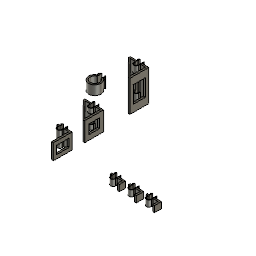
EinklickbareHalterungen (Autodesk Fusion 360 design; units mm, degrees)
part number: 2025-11-29-23-14-23-792
Autodesk Fusion 360 part; units mm, degrees
note: some values were not read from the file. Chosen so that the rebuilt part matches the saved one: which bodies a step acts on; which face or edge a step refers to. Set by a fixed rule: which sketch regions a step uses.
sketch "Skizze1" plane through (0, 0, 0) normal (0, 0, 1) x (1, 0, 0)
  line L0 (0, 0) -> (50, 0)
  line L1 (50, 0) -> (50, 25)
  line L2 (50, 25) -> (0, 25)
  line L3 (0, 25) -> (0, 0)
  line L4 (38.3, 22) -> (11.7, 22)
  line L5 (11.7, 22) -> (11.7, 3)
  line L6 (11.7, 3) -> (38.3, 3)
  line L7 (38.3, 3) -> (38.3, 22)
  line L8 (38.3, 22) -> (11.7, 3) construction
  line L9 (11.7, 22) -> (38.3, 3) construction
  point P0 (25, 12.5)
  dimension "d1" = 50
  dimension "d2" = 25
  dimension "d3" = 26.6
  dimension "d4" = 19
  constraint horizontal L0
  constraint vertical L1
  constraint horizontal L2
  constraint vertical L3
  constraint coincident L0.start L3.end
  constraint horizontal L4
  constraint perpendicular L4 L5
  constraint parallel L4 L6
  constraint parallel L5 L7
  constraint coincident L8 P0
  constraint coincident L9 P0
  measures "d1" distance of L0.start L0.end
  measures "d2" distance of L0.start L2.end
  measures "d3" distance of L5.end L6.end
  measures "d4" distance of L4.end L5.end
extrude "Extrusion1" add sketch "Skizze1" along normal blind 2 makes body 1
sketch "Skizze2" plane through (0, 0, 2) normal (0, 0, 1) x (-1, 0, 0)
  line L0 (-38.3, -22) -> (-38.3, -3)
  line L1 (-38.3, -3) -> (-11.7, -3)
  line L2 (-11.7, -3) -> (-11.7, -22)
  line L3 (-11.7, -22) -> (-38.3, -22)
  line L4 (0, -25) -> (0, 0)
  line L5 (0, 0) -> (-50, 0)
  line L6 (-50, 0) -> (-50, -25)
  line L7 (-50, -25) -> (0, -25)
  line L8 (-11.7, -12.5) -> (-5, -12.5)
  line L9 (-38.3, -12.5) -> (-45, -12.5)
  circle A0 centre (-5, -12.5) radius 1.35
  circle A1 centre (-45, -12.5) radius 1.35
  dimension "d7" = 6.7
  dimension "d8" = 6.7
  dimension "d9" = 2.7
  dimension "d10" = 2.7
  constraint midpoint L2 L8.start
  constraint perpendicular L0 L8
  constraint midpoint L0 L9.start
  constraint perpendicular L0 L9
  constraint coincident L8.end A0.centre
  constraint coincident L9.end A1.centre
  measures "d7" distance of L8.start L8.end
  measures "d8" distance of L9.start L9.end
  measures "d9" diameter of A0
  measures "d10" diameter of A1
sketch "Skizze3" plane through (0, 0, 0) normal (0, 1, 0) x (1, 0, 0)
sketch "Skizze4" plane through (0, 0, 2) normal (0, 0, 1) x (-1, 0, 0)
  line L0 (-38.3, -22) -> (-38.3, -3)
  line L1 (-38.3, -3) -> (-11.7, -3)
  line L2 (-11.7, -3) -> (-11.7, -22)
  line L3 (-11.7, -22) -> (-38.3, -22)
  line L4 (0, -25) -> (0, 0)
  line L5 (0, 0) -> (-50, 0)
  line L6 (-50, 0) -> (-50, -25)
  line L7 (-50, -25) -> (0, -25)
  line L8 (-110, 0) -> (-80, 0)
  line L9 (-80, 0) -> (-80, -25)
  line L10 (-80, -25) -> (-110, -25)
  line L11 (-110, -25) -> (-110, 0)
  dimension "d13" = 30
  dimension "d14" = 25
  constraint horizontal L8
  constraint vertical L9
  constraint horizontal L10
  constraint vertical L11
  measures "d13" distance of L8.start L8.end
  measures "d14" distance of L8.start L10.end
sketch "Skizze5" plane through (0, 0, 1) normal (0, 0, 1) x (-1, 0, 0)
  line L0 (-110, -25) -> (-80, -25)
  line L1 (-80, -25) -> (-80, 0)
  line L2 (-80, 0) -> (-110, 0)
  line L3 (-110, 0) -> (-110, -25)
  line L4 (-80, 0) -> (-110, -25) construction
  line L5 (-110, 0) -> (-80, -25) construction
  line L6 (-102.25, -20.5) -> (-87.75, -20.5)
  line L7 (-87.75, -20.5) -> (-87.75, -4.5)
  line L8 (-87.75, -4.5) -> (-102.25, -4.5)
  line L9 (-102.25, -4.5) -> (-102.25, -20.5)
  line L10 (-102.25, -20.5) -> (-87.75, -4.5) construction
  line L11 (-87.75, -20.5) -> (-102.25, -4.5) construction
  point P0 (-95, -12.5)
  dimension "d17" = 14.5
  dimension "d18" = 16
  constraint coincident L1.end L2.start
  constraint coincident L0.start L3.end
  constraint coincident L2.end L3.start
  constraint coincident L0.end L1.start
  constraint horizontal L6
  constraint perpendicular L6 L7
  constraint parallel L6 L8
  constraint parallel L7 L9
  constraint coincident L10 P0
  constraint coincident L11 P0
  constraint midpoint L4 P0
  measures "d17" distance of L7.end L8.end
  measures "d18" distance of L6.end L7.end
move_body "Verschieben2" [no effect]
sketch "Skizze6" plane through (0, 0, 0) normal (-1, 0, 0) x (0, -1, 0)
  line L0 (-25, 0) -> (0, 0)
  line L1 (0, 0) -> (0, 2)
  line L2 (0, 2) -> (-25, 2)
  line L3 (-25, 2) -> (-25, 0)
  line L4 (-25, 0) -> (-25, 10.9)
  line L5 (-25, 0) -> (-23.5, 0)
  line L6 (-23.5, 0) -> (-23.5, 30)
  line L7 (-23.5, 30) -> (-25, 30)
  line L8 (-25, 30) -> (-25, 0)
  line L9 (-25, 30) -> (-25, 19.1)
  line L10 (-25, 10.9) -> (-25, 11.9)
  line L11 (-25, 19.1) -> (-25, 18.1)
  line L12 (-25, 11.9) -> (-25, 18.1)
  line L13 (-25, 0) -> (-25, 11)
  line L14 (-25, 30) -> (-25, 19)
  line L15 (-25, 19) -> (-27.3, 19)
  line L16 (-27.3, 19) -> (-27.3, 20.5)
  line L17 (-25, 10.9) -> (-25, 11.65)
  line L18 (-27.3, 9.4) -> (-24.118, 9.4) construction
  line L19 (-25, 19) -> (-25, 18.25)
  line L20 (-27.3, 20.5) -> (-29.55, 18.25)
  line L21 (-27.3, 20.5) -> (-24.118, 20.5) construction
  line L22 (-29.55, 18.25) -> (-25, 18.25)
  line L23 (-25, 30) -> (-25, 22)
  line L24 (-25, 22) -> (-23.5, 22)
  line L25 (-25, 15) -> (-20, 15) construction
  line L26 (-25, 18.25) -> (-20, 18.25)
  line L27 (-25, 19) -> (-20, 19)
  line L28 (-25, 0) -> (-25, 11)
  line L29 (-25, 11) -> (-27.3, 11)
  line L30 (-27.3, 11) -> (-27.3, 9.5)
  line L31 (-25, 11) -> (-25, 11.75)
  line L32 (-27.3, 9.5) -> (-29.5511, 11.75)
  line L33 (-29.5511, 11.75) -> (-25, 11.75)
  circle A0 centre (-20, 15) radius 3.25
  line L34 (-25, 11) -> (-20, 11)
  line L35 (-25, 11.75) -> (-20, 11.75)
  circle A1 centre (-20, 15) radius 4
  dimension "d29" = 10.9
  dimension "d30" = 1.5
  dimension "d31" = 30
  dimension "d32" = 10.9
  dimension "d42" = 1
  dimension "d43" = 1
  dimension "d52" = 11
  dimension "d53" = 2.3
  dimension "d54" = 1.5
  dimension "d56" = 0.75
  dimension "d58" = 0.75
  dimension "d59" = 135
  dimension "d61" = 1.5
  dimension "d62" = 0.75
  constraint coincident L0.start L3.end
  constraint perpendicular L2 L4
  constraint horizontal L5
  constraint vertical L6
  constraint horizontal L7
  constraint vertical L8
  constraint perpendicular L7 L9
  constraint coincident L10 L13.end
  constraint parallel L10 L13
  constraint perpendicular L7 L14
  constraint perpendicular L14 L15
  constraint perpendicular L15 L16
  constraint horizontal L18
  constraint perpendicular L15 L19
  constraint horizontal L21
  constraint perpendicular L8 L22
  constraint coincident L14 L23.end
  constraint coincident L6 L24.end
  constraint perpendicular L6 L24
  constraint midpoint L12 L25.start
  constraint perpendicular L12 L25
  constraint perpendicular L11 L26
  constraint perpendicular L8 L27
  constraint perpendicular L16 L29
  constraint perpendicular L18 L30
  constraint perpendicular L29 L31
  constraint perpendicular L8 L33
  constraint coincident L25.end A0.centre
  constraint coincident L26.end A0
  constraint tangent L26 A0
  constraint perpendicular L17 L34
  constraint coincident A0 L35.end
  constraint tangent A0 L35
  constraint coincident L27.end A1
  constraint tangent L27 A1
  measures "d29" distance of L0.start L4.end
  measures "d30" distance of L0.start L5.end
  measures "d31" distance of L0.start L7.end
  measures "d32" distance of L7.end L9.end
  measures "d42" distance of L4.end L10.end
  measures "d43" distance of L9.end L11.end
  measures "d52" distance of L7.end L14.end
  measures "d53" distance of L14.end L15.end
  measures "d54" distance of L15.end L16.end
  measures "d56" distance of L4.end L17.end
  measures "d58" distance of L14.end L19.end
  measures "d59" angle of L20 L21
  measures "d61" distance of L29.end L30.end
  measures "d62" distance of L13.end L31.end
extrude "Extrusion12" add sketch "Skizze6" against normal blind 50 contours L2 L4 L6 L8 L10 L13 L17 L28 L34 | L6 L8 L10 L17 L31 L34 L35 | L6 L34 L35 A1 | L8 L10 L17 L29 L30 L31 L32 L33 | L26 A0 L35 A1 | L6 L26 L27 A1 | L6 L8 L11 L19 L26 L27 | L6 L8 L9 L11 L14 L24 L27 | L8 L11 L15 L16 L19 L20 L22 bodies 1
move_body "Verschieben5" bodies 1 to x (0, 0, 1) y (0, 1, 0) z (-1, 0, 0) at (0, 0, 0)
sketch "Skizze7" plane through (0, 0, 0) normal (0, 0, 1) x (1, 0, 0)
  circle A0 centre (55, 0) radius 7.5
  circle A1 centre (55, 0) radius 10
  line L0 (55, 0) -> (58, 0)
  line L1 (58, 0) -> (52, 0)
  line L2 (52, 0) -> (52, 20)
  line L3 (52, 20) -> (58, 20)
  line L4 (58, 20) -> (58, 0)
  line L5 (55, 0) -> (59.7, 0)
  line L6 (59.7, 0) -> (50.3, 0)
  line L7 (50.3, 0) -> (50.3, 20)
  line L8 (50.3, 20) -> (59.7, 20)
  line L9 (59.7, 20) -> (59.7, 0)
  line L10 (50.3, 8.8267) -> (50.3, 11.0767)
  line L11 (59.7, 8.8267) -> (59.7, 11.0767)
  line L12 (59.7, 11.0767) -> (61.38, 11.0767)
  line L13 (50.3, 11.0767) -> (48.62, 11.0767)
  line L14 (48.62, 11.0767) -> (52, 14.4567)
  line L15 (48.62, 11.0767) -> (53.4, 11.0767) construction
  line L16 (61.38, 11.0767) -> (58, 14.4567)
  dimension "d66" = 15
  dimension "d67" = 20
  dimension "d68" = 6
  dimension "d69" = 20
  dimension "d71" = 9.4
  dimension "d72" = 20
  dimension "d73" = 2.25
  dimension "d74" = 2.25
  dimension "d75" = 1.68
  dimension "d76" = 1.68
  dimension "d77" = 45
  constraint concentric A0 A1
  constraint coincident A0.centre A1.centre
  constraint horizontal L0
  constraint horizontal L1
  constraint vertical L2
  constraint horizontal L3
  constraint vertical L4
  constraint perpendicular L4 L5
  constraint horizontal L6
  constraint vertical L7
  constraint horizontal L8
  constraint vertical L9
  constraint coincident A1 L10.start
  constraint coincident L7 L10.start
  constraint parallel L7 L10
  constraint coincident A1 L11.start
  constraint coincident L9 L11.start
  constraint parallel L9 L11
  constraint perpendicular L11 L12
  constraint perpendicular L7 L13
  constraint horizontal L15
  constraint coincident L2 L14.end
  constraint coincident L4 L16.end
  constraint perpendicular L14 L16
  measures "d66" diameter of A0
  measures "d67" diameter of A1
  measures "d68" distance of L0.end L1.end
  measures "d69" distance of L1 L3
  measures "d71" distance of L5.end L6.end
  measures "d72" distance of L5.end L8.end
  measures "d73" distance of L10.start L10.end
  measures "d74" distance of L11.start L11.end
  measures "d75" distance of L11.end L12.end
  measures "d76" distance of L10.end L13.end
  measures "d77" angle of L14 L15
extrude "Extrusion13" add sketch "Skizze7" along normal blind 2 separate body contours A0 A1 L7 L9 | A0 A1 L4 L9 | A0 A1 L2 L7 | A1 L4 L9 L11 L16 | A1 L2 L7 L10 L14 | L9 L12 L16 | L7 L13 L14 makes body 2
extrude "Extrusion14" add 1 faces at (51.4333, 12.2509, 2) along direction (0, 0, 1) blind 3 on bodies 2 bodies 2
sketch "Skizze8" plane through (0, 0, 0) normal (0, 0, 1) x (1, 0, 0)
  line L0 (55, 0) -> (70, 0)
  line L1 (59.7, 8.8267) -> (59.7, 11.0767)
  arc A0 (50.3, 8.8267) -> (59.7, 8.8267) centre (55, 0) ccw
  line L2 (59.7, 8.8267) -> (70, 8.8267)
  line L3 (70, 8.8267) -> (70, -16.1733)
  line L4 (70, 8.8267) -> (68, 8.8267)
  line L5 (68, 8.8267) -> (68, -16.1733)
  line L6 (68, -16.1733) -> (70, -16.1733)
  line L7 (70, -16.1733) -> (70, 8.8267)
  line L8 (68, 0) -> (64.1652, 0)
  line L9 (64.1652, 0) -> (64.1652, 4)
  line L10 (64.1652, 4) -> (68, 4)
  line L11 (68, 4) -> (68, 0)
  line L12 (68, 0) -> (64.1652, 0)
  line L13 (64.1652, 0) -> (64.1652, -4)
  line L14 (64.1652, -4) -> (68, -4)
  line L15 (68, -4) -> (68, 0)
  dimension "d82" = 15
  dimension "d83" = 25
  dimension "d84" = 2
  dimension "d85" = 25
  dimension "d86" = 4
  dimension "d87" = 4
  constraint horizontal L0
  constraint coincident L1.start A0.end
  constraint perpendicular L1 L2
  constraint perpendicular L2 L3
  constraint horizontal L4
  constraint vertical L5
  constraint horizontal L6
  constraint vertical L7
  constraint horizontal L8
  constraint vertical L9
  constraint horizontal L10
  constraint vertical L11
  constraint coincident A0 L9.end
  constraint coincident L0 L8.start
  constraint horizontal L12
  constraint vertical L13
  constraint horizontal L14
  constraint vertical L15
  constraint coincident A0 L13.end
  measures "d82" distance of L0.start L0.end
  measures "d83" distance of L2.end L3.end
  measures "d84" distance of L2.end L4.end
  measures "d85" distance of L2.end L3.end
  measures "d86" distance of L8.start L10.end
  measures "d87" distance of L8.start L14.end
extrude "Extrusion15" add sketch "Skizze8" along normal blind 5 contours L0 L2 L3 L4 L5 L7 L11 | L0 A0 L5 L8 L12 L14 L15 | L0 A0 L5 L8 L10 L11 L12 | L0 L3 L5 L6 L7 L15 bodies 2
extrude "Extrusion16" add 1 faces at (66.1661, -0.0532, 5) along direction (0, 0, 1) blind 5 on bodies 2 bodies 2
extrude "Extrusion17" add 1 faces at (66.1661, -0.0532, 10) along direction (0, 0, 1) blind 1.7 on bodies 2 bodies 2
sketch "Skizze10" plane through (0, 0, 11.7) normal (0, 0, 1) x (-1, 0, 0)
  arc A0 (-50.3, -8.8267) -> (-64.1652, 4) centre (-55, 0) ccw
  line L0 (-64.1652, 4) -> (-68, 4)
  line L1 (-68, 4) -> (-68, 16.1733)
  line L2 (-68, 16.1733) -> (-70, 16.1733)
  line L3 (-70, 16.1733) -> (-70, -8.8267)
  line L4 (-70, -8.8267) -> (-68, -8.8267)
  line L5 (-68, -8.8267) -> (-68, -4)
  line L6 (-68, -4) -> (-64.1652, -4)
  arc A1 (-64.1652, -4) -> (-59.7, -8.8267) centre (-55, 0) ccw
  line L7 (-59.7, -8.8267) -> (-59.7, -11.0767)
  line L8 (-59.7, -11.0767) -> (-61.38, -11.0767)
  line L9 (-61.38, -11.0767) -> (-58, -14.4567)
  line L10 (-58, -14.4567) -> (-58, -6.8739)
  arc A2 (-52, -6.8739) -> (-58, -6.8739) centre (-55, 0) ccw
  line L11 (-52, -6.8739) -> (-52, -14.4567)
  line L12 (-52, -14.4567) -> (-48.62, -11.0767)
  line L13 (-48.62, -11.0767) -> (-50.3, -11.0767)
  line L14 (-50.3, -11.0767) -> (-50.3, -8.8267)
  line L15 (-70, -8.8267) -> (-68, -8.8267)
  line L16 (-68, -8.8267) -> (-68, 16.1733)
  line L17 (-68, 16.1733) -> (-70, 16.1733)
  line L18 (-70, 16.1733) -> (-70, -8.8267)
  constraint horizontal L15
  constraint vertical L16
  constraint horizontal L17
  constraint vertical L18
  constraint coincident L1.end L2.start
  constraint coincident L3.end L4.start
extrude "Extrusion18" add sketch "Skizze10" along normal blind 26.6 contours L1 L2 L3 L4 L5 L15 L16 L17 L18 bodies 2
extrude "Extrusion19" add 1 faces at (66.1661, -0.0532, 0) along direction (0, 0, 1) blind 11.7 from surface at 38.3 on bodies 2 bodies 2
sketch "Skizze11" plane through (70, 0, 0) normal (1, 0, 0) x (0, 1, 0)
  line L0 (-16.1733, 0) -> (8.8267, 0)
  line L1 (8.8267, 0) -> (8.8267, 50)
  line L2 (8.8267, 50) -> (-16.1733, 50)
  line L3 (-16.1733, 50) -> (-16.1733, 0)
  line L4 (-16.1733, 50) -> (8.8267, 0) construction
  line L5 (-16.1733, 0) -> (8.8267, 50) construction
  line L6 (5.8267, 38.3) -> (-13.1733, 38.3)
  line L7 (-13.1733, 38.3) -> (-13.1733, 11.7)
  line L8 (-13.1733, 11.7) -> (5.8267, 11.7)
  line L9 (5.8267, 11.7) -> (5.8267, 38.3)
  line L10 (5.8267, 38.3) -> (-13.1733, 11.7) construction
  line L11 (-13.1733, 38.3) -> (5.8267, 11.7) construction
  point P0 (-3.6733, 25)
  dimension "d99" = 19
  dimension "d100" = 26.6
  constraint coincident L2.end L3.start
  constraint coincident L0.end L1.start
  constraint coincident L0.start L3.end
  constraint coincident L1.end L2.start
  constraint horizontal L6
  constraint perpendicular L6 L7
  constraint parallel L6 L8
  constraint parallel L7 L9
  constraint coincident L10 P0
  constraint coincident L11 P0
  constraint midpoint L5 P0
  measures "d99" distance of L7.end L8.end
  measures "d100" distance of L6.end L7.end
extrude "Extrusion20" cut sketch "Skizze11" against normal blind 8 contours L6 L7 L8 L9 bodies 2
split "Teilen1" by plane through (70, -13.1733, 11.7) normal (0, 0, 1) bodies 2 makes body 3 at (57.0044, -7.2272, 46.1)
combine "Kombinieren1" operation add target body 2 tool bodies 3
sketch "Skizze12" plane through (0, 0, 0) normal (0, 0, 1) x (1, 0, 0)
  line L0 (-56.3, 20) -> (-56.3, 0)
  line L1 (-65.7, 0) -> (-65.7, 20)
  line L2 (-65.7, 8.8267) -> (-65.7, 11.0767)
  line L3 (-64, 0) -> (-64, 20)
  line L4 (-67.38, 11.0767) -> (-62.6, 11.0767) construction
  circle A0 centre (-61, 0) radius 7.5
  line L5 (-64, 20) -> (-58, 20)
  line L6 (-67.38, 11.0767) -> (-64, 14.4567)
  line L7 (-56.3, 11.0767) -> (-54.62, 11.0767)
  line L8 (-54.62, 11.0767) -> (-58, 14.4567)
  line L9 (-58, 0) -> (-64, 0)
  line L10 (-56.3, 8.8267) -> (-56.3, 11.0767)
  line L11 (-65.7, 11.0767) -> (-67.38, 11.0767)
  line L12 (-61, 0) -> (-58, 0)
  line L13 (-61, 0) -> (-56.3, 0)
  circle A1 centre (-61, 0) radius 10
  line L14 (-56.3, 0) -> (-65.7, 0)
  line L15 (-58, 20) -> (-58, 0)
  line L16 (-65.7, 20) -> (-56.3, 20)
  dimension "d103" = 15
  dimension "d104" = 20
  dimension "d105" = 6
  dimension "d106" = 20
  dimension "d107" = 9.4
  dimension "d108" = 20
  dimension "d109" = 2.25
  dimension "d110" = 2.25
  dimension "d111" = 1.68
  dimension "d112" = 1.68
  dimension "d113" = 45
  constraint concentric A0 A1
  constraint coincident A0.centre L12.start
  constraint horizontal L12
  constraint horizontal L9
  constraint vertical L3
  constraint horizontal L5
  constraint vertical L15
  constraint perpendicular L13 L15
  constraint horizontal L14
  constraint vertical L1
  constraint horizontal L16
  constraint vertical L0
  constraint coincident L2.start A1
  constraint coincident L2.start L1
  constraint parallel L1 L2
  constraint coincident L10.start A1
  constraint coincident L10.start L0
  constraint parallel L0 L10
  constraint perpendicular L7 L10
  constraint perpendicular L1 L11
  constraint horizontal L4
  constraint coincident L6.end L3
  constraint coincident L8.end L15
  constraint perpendicular L6 L8
  measures "d103" diameter of A0
  measures "d104" diameter of A1
  measures "d105" distance of L9.start L3.start
  measures "d106" distance of L5 L9
  measures "d107" distance of L1.start L0.end
  measures "d108" distance of L0.end L0.start
  measures "d109" distance of L2.end L2.start
  measures "d110" distance of L10.start L7.start
  measures "d111" distance of L7.end L7.start
  measures "d112" distance of L2.end L4.start
  measures "d113" angle of L4 L6
extrude "Extrusion21" add sketch "Skizze12" along normal blind 5 separate body contours L0 L8 L10 A1 L15 | L0 L7 L8 | L0 L1 A0 A1 | L0 A0 A1 L15 | L1 L3 A0 A1 | L1 L2 L3 L6 A1 | L1 L6 L11 makes body 4
sketch "Skizze13" plane through (0, 0, 0) normal (0, 0, 1) x (1, 0, 0)
  line L0 (15.3, 8.8267) -> (15.3, 11.0767)
  line L1 (13.62, 11.0767) -> (18.4, 11.0767) construction
  circle A0 centre (20, 0) radius 7.5
  line L2 (13.62, 11.0767) -> (17, 14.4567)
  line L3 (24.7, 11.0767) -> (26.38, 11.0767)
  line L4 (26.38, 11.0767) -> (23, 14.4567)
  line L5 (24.7, 8.8267) -> (24.7, 11.0767)
  line L6 (15.3, 11.0767) -> (13.62, 11.0767)
  circle A1 centre (20, 0) radius 10
  line L7 (35, 0) -> (35, 8.8267)
  line L8 (35, 8.8267) -> (33, 8.8267)
  line L9 (33, -16.1733) -> (35, -16.1733)
  line L10 (35, -16.1733) -> (35, 8.8267)
  line L11 (29.1652, 4) -> (33, 4)
  line L12 (29.1652, -4) -> (33, -4)
  line L13 (17, 14.4567) -> (17, 9.5394)
  line L14 (23, 14.4567) -> (23, 9.5394)
  line L15 (23, 9.5394) -> (23, 6.8739)
  line L16 (17, 9.5394) -> (17, 6.8739)
  line L17 (33, 4) -> (33, 8.8267)
  line L18 (33, -4) -> (33, -16.1733)
  dimension "d116" = 15
  dimension "d117" = 20
  dimension "d122" = 2.25
  dimension "d123" = 2.25
  dimension "d124" = 1.68
  dimension "d125" = 1.68
  dimension "d126" = 45
  dimension "d127" = 2
  dimension "d128" = 25
  dimension "d131" = 135
  dimension "d132" = 6
  dimension "d133" = 9.4
  dimension "d134" = 12.76
  constraint concentric A0 A1
  constraint coincident L0.start A1
  constraint coincident L5.start A1
  constraint perpendicular L3 L5
  constraint horizontal L1
  constraint perpendicular L2 L4
  constraint horizontal L8
  constraint horizontal L9
  constraint vertical L10
  constraint horizontal L11
  constraint coincident A1 L11.start
  constraint horizontal L12
  constraint coincident A1 L12.start
  constraint coincident A1 L13.end
  constraint perpendicular L1 L13
  constraint coincident A1 L14.end
  constraint parallel L13 L14
  constraint coincident A0 L15.end
  constraint parallel L14 L15
  constraint coincident A0 L16.end
  constraint parallel L13 L16
  measures "d116" diameter of A0
  measures "d117" diameter of A1
  measures "d122" distance of L0.end L0.start
  measures "d123" distance of L5.start L3.start
  measures "d124" distance of L3.end L3.start
  measures "d125" distance of L0.end L1.start
  measures "d126" angle of L1 L2
  measures "d127" distance of L7.end L8.end
  measures "d128" distance of L7.end L9.end
  measures "d131" angle of L3 L4
  measures "d132" distance of L13 L14
  measures "d133" distance of L0 L5
  measures "d134" distance of L3.end L1.start
copy_body "Körper kopieren/einfügen3" bodies 1 makes body 5
move_body "Verschieben7" bodies 5 to x (1, 0, 0) y (0, 1, 0) z (0, 0, 1) at (0, -72, 0)
sketch "Skizze14" plane through (0, 0, 0) normal (1, 0, 0) x (0, 1, 0)
  line L0 (-69, 38.3) -> (-50, 38.3)
  line L1 (-50, 38.3) -> (-50, 11.7)
  line L2 (-50, 11.7) -> (-69, 11.7)
  line L3 (-69, 11.7) -> (-69, 38.3)
  line L4 (-72, 0) -> (-47, 0)
  line L5 (-47, 0) -> (-47, 50)
  line L6 (-47, 50) -> (-72, 50)
  line L7 (-72, 50) -> (-72, 0)
extrude "Extrusion22" add sketch "Skizze14" against normal blind 2 contours L0 L1 L2 L3 bodies 5
sketch "Skizze15" plane through (0, 0, 0) normal (1, 0, 0) x (0, 1, 0)
  line L0 (-72, 0) -> (-47, 0)
  line L1 (-47, 0) -> (-47, 50)
  line L2 (-47, 50) -> (-72, 50)
  line L3 (-72, 50) -> (-72, 0)
  line L4 (-59.5, 0) -> (-59.5, 5)
  line L5 (-59.5, 5) -> (-51.5, 5)
  line L6 (-51.5, 5) -> (-67.5, 5)
  line L7 (-67.5, 5) -> (-67.5, 19.5)
  line L8 (-67.5, 19.5) -> (-51.5, 19.5)
  line L9 (-51.5, 19.5) -> (-51.5, 5)
  dimension "d137" = 5
  dimension "d138" = 8
  dimension "d139" = 16
  dimension "d140" = 14.5
  constraint midpoint L0 L4.start
  constraint perpendicular L0 L4
  constraint perpendicular L4 L5
  constraint horizontal L6
  constraint vertical L7
  constraint horizontal L8
  constraint vertical L9
  measures "d137" distance of L4.start L4.end
  measures "d138" distance of L4.end L5.end
  measures "d139" distance of L5.end L6.end
  measures "d140" distance of L5.end L8.end
extrude "Extrusion23" cut 1 faces at (-0.6667, -55.8333, 50) along direction (0, 0, -1) blind 25.5 on bodies 5 bodies 5
extrude "Extrusion24" cut sketch "Skizze15" against normal blind 2 contours L5 L6 L7 L8 L9 bodies 5
sketch "Skizze16" plane through (0, 0, 0) normal (0, 0, 1) x (1, 0, 0)
  line L0 (-210.8348, -136) -> (-207, -136)
  line L1 (-223, -125.5433) -> (-223, -130.4606)
  line L2 (-205, -140) -> (-205, -131.1733)
  line L3 (-223, -130.4606) -> (-223, -133.1261)
  line L4 (-213.62, -128.9233) -> (-217, -125.5433)
  line L5 (-224.7, -128.9233) -> (-226.38, -128.9233)
  line L6 (-226.38, -128.9233) -> (-221.6, -128.9233) construction
  circle A0 centre (-220, -140) radius 10
  line L7 (-207, -144) -> (-207, -156.1733)
  line L8 (-205, -156.1733) -> (-205, -131.1733)
  circle A1 centre (-220, -140) radius 7.5
  line L9 (-224.7, -131.1733) -> (-224.7, -128.9233)
  line L10 (-205, -131.1733) -> (-207, -131.1733)
  line L11 (-207, -156.1733) -> (-205, -156.1733)
  line L12 (-217, -130.4606) -> (-217, -133.1261)
  line L13 (-226.38, -128.9233) -> (-223, -125.5433)
  line L14 (-210.8348, -144) -> (-207, -144)
  line L15 (-215.3, -128.9233) -> (-213.62, -128.9233)
  line L16 (-207, -136) -> (-207, -131.1733)
  line L17 (-215.3, -131.1733) -> (-215.3, -128.9233)
  line L18 (-217, -125.5433) -> (-217, -130.4606)
  dimension "d145" = 15
  dimension "d146" = 20
  dimension "d147" = 2.25
  dimension "d148" = 2.25
  dimension "d149" = 1.68
  dimension "d150" = 1.68
  dimension "d151" = 45
  dimension "d152" = 2
  dimension "d153" = 25
  dimension "d154" = 135
  dimension "d155" = 6
  dimension "d156" = 9.4
  dimension "d157" = 12.76
  constraint concentric A0 A1
  constraint coincident L9.start A0
  constraint coincident L17.start A0
  constraint perpendicular L15 L17
  constraint horizontal L6
  constraint perpendicular L4 L13
  constraint horizontal L10
  constraint horizontal L11
  constraint vertical L8
  constraint horizontal L0
  constraint coincident L0.start A0
  constraint horizontal L14
  constraint coincident L14.start A0
  constraint coincident L1.end A0
  constraint perpendicular L1 L6
  constraint coincident L12.start A0
  constraint parallel L1 L18
  constraint coincident L12.end A1
  constraint parallel L12 L18
  constraint coincident L3.end A1
  constraint parallel L1 L3
  measures "d145" diameter of A1
  measures "d146" diameter of A0
  measures "d147" distance of L5.start L9.start
  measures "d148" distance of L17.start L15.start
  measures "d149" distance of L4.start L15.start
  measures "d150" distance of L5.end L5.start
  measures "d151" angle of L6 L13
  measures "d152" distance of L10.end L2.end
  measures "d153" distance of L8.start L2.end
  measures "d154" angle of L4 L15
  measures "d155" distance of L1 L18
  measures "d156" distance of L9 L17
  measures "d157" distance of L5.end L4.start
extrude "Extrusion25" add sketch "Skizze13" along normal blind 10 separate body contours L0 L2 L6 A1 L13 | A0 A1 L15 L16 | A1 L7 L8 L9 L10 L11 L12 L17 L18 | L3 L4 L5 A1 L14 picked at (13.0908, 5.9969) makes body 6
extrude "Extrusion26" add 1 faces at (31.8333, -1.3333, 10) along direction (0, 0, 1) blind 100 on bodies 6 bodies 6
extrude "Extrusion27" cut 1 faces at (31.1661, -0.0532, 110) along direction (0, 0, -1) blind 110 on bodies 6 bodies 6
extrude "Extrusion28" add sketch "Skizze13" along normal blind 110 contours L0 L2 L6 A1 L13 | A0 A1 L15 L16 | A1 L7 L8 L9 L10 L11 L12 L17 L18 | L3 L4 L5 A1 L14 picked at (13.0908, 5.9969) bodies 6
extrude "Extrusion29" cut 1 faces at (31.8333, -1.3333, 110) along direction (0, 0, -1) blind 110 on bodies 6 bodies 6
extrude "Extrusion30" add sketch "Skizze13" along normal blind 25.5 contours L0 L2 L6 A1 L13 | A0 A1 L15 L16 | A1 L7 L8 L9 L10 L11 L12 L17 L18 | L3 L4 L5 A1 L14 picked at (13.0908, 5.9969) bodies 6
extrude "Extrusion31" add 1 faces at (-64.5667, 12.2509, 5) along direction (0, 0, 1) blind 10 on bodies 4 bodies 4
extrude "Extrusion32" cut 1 faces at (-1.3333, -62.1667, 5) along direction (0, 0, -1) blind 0.1 on bodies 5 bodies 5
extrude "Extrusion33" cut 1 faces at (-1.3333, -62.1667, 19.5) along direction (0, 0, 1) blind 0.1 on bodies 5 bodies 5
extrude "Extrusion34" cut 1 faces at (-1.3333, -67.5, 14.7) along direction (0, -1, 0) blind 0.1 on bodies 5 bodies 5
extrude "Extrusion35" cut 1 faces at (-0.6667, -51.5, 9.8) along direction (0, 1, 0) blind 0.1 on bodies 5 bodies 5
sketch "Skizze17" plane through (-19, 0, 0) normal (-1, 0, 0) x (0, -1, 0)
  line L0 (52, 24.5) -> (48.5, 24.5)
  line L1 (48.5, 24.5) -> (48.5, 0)
  line L2 (48.5, 0) -> (52, 0)
  line L3 (52, 0) -> (52, 24.5)
  line L4 (48.5, 0) -> (48.5, 4.9)
  line L5 (48.5, 4.9) -> (56.261, 4.9)
  line L6 (56.261, 4.9) -> (56.261, 19.6)
  line L7 (56.261, 19.6) -> (48.5, 19.6)
  line L8 (48.5, 19.6) -> (48.5, 4.9)
  dimension "d180" = 4.9
  dimension "d181" = 14.7
  constraint coincident L1.end L2.start
  constraint perpendicular L2 L4
  constraint horizontal L5
  constraint vertical L6
  constraint horizontal L7
  constraint vertical L8
  measures "d180" distance of L1.end L4.end
  measures "d181" distance of L4.end L7.end
extrude "Extrusion36" cut sketch "Skizze17" against normal blind 15 contours L3 L5 L6 L7 | L1 L3 L5 L7 L8 bodies 5
extrude "Extrusion37" add 1 faces at (-0.6667, -55.8333, 0) along direction (0, 0, -1) blind 3 on bodies 5 bodies 5
extrude "Extrusion38" add 1 faces at (-0.6667, -55.8333, 24.5) along direction (0, 0, 1) blind 3 on bodies 5 bodies 5
extrude "Extrusion39" cut 1 faces at (-0.6667, 15.6667, 11.7) along direction (0, 0, -1) blind 0.1 on bodies 1 bodies 1
extrude "Extrusion40" cut 1 faces at (-0.6667, 9.3333, 38.3) along direction (0, 0, 1) blind 0.1 on bodies 1 bodies 1
extrude "Extrusion41" cut 1 faces at (-0.6667, 22, 20.5333) along direction (0, 1, 0) blind 0.1 on bodies 1 bodies 1
extrude "Extrusion42" cut 1 faces at (-0.6667, 3, 20.5333) along direction (0, -1, 0) blind 0.1 on bodies 1 bodies 1
sketch "Skizze18" plane through (-19, 0, 0) normal (-1, 0, 0) x (0, -1, 0)
  line L0 (-23.5, 0) -> (-20, 0)
  line L1 (-20, 0) -> (-20, 50)
  line L2 (-20, 50) -> (-23.5, 50)
  line L3 (-23.5, 50) -> (-23.5, 0)
  line L4 (-23.5, 0) -> (-23.5, 11.6)
  line L5 (-23.5, 11.6) -> (-15, 11.6)
  line L6 (-15, 11.6) -> (-15, 38.4)
  line L7 (-15, 38.4) -> (-23.5, 38.4)
  line L8 (-23.5, 38.4) -> (-23.5, 11.6)
  dimension "d196" = 11.6
  dimension "d197" = 26.8
  constraint coincident L0.start L3.end
  constraint perpendicular L0 L4
  constraint horizontal L5
  constraint vertical L6
  constraint horizontal L7
  constraint vertical L8
  measures "d196" distance of L0.start L4.end
  measures "d197" distance of L4.end L7.end
extrude "Extrusion43" cut sketch "Skizze18" against normal blind 11 contours L1 L3 L5 L7 L8 | L1 L5 L6 L7 bodies 1
extrude "Extrusion44" add 1 faces at (-2, -62.7, -0.3667) along direction (-1, 0, 0) blind 1 on bodies 5 bodies 5
extrude "Extrusion45" add 1 faces at (-5.6667, -48.5, 9.8) along direction (0, -1, 0) blind 1 on bodies 5 bodies 5
extrude "Extrusion46" add 1 faces at (-21, -48.5, 14.7) along direction (0, -1, 0) blind 1 on bodies 5 bodies 5
extrude "Extrusion47" add 1 faces at (-2, 8.8, 46.1333) along direction (-1, 0, 0) blind 1 on bodies 1 bodies 1
extrude "Extrusion48" add 1 faces at (-5.6667, 23.5, 29.4667) along direction (0, -1, 0) blind 1 on bodies 1 bodies 1
extrude "Extrusion49" add 1 faces at (-21, 23.5, 29.4667) along direction (0, -1, 0) blind 1 on bodies 1 bodies 1
copy_body "Körper kopieren/einfügen4" bodies 5 makes body 7
move_body "Verschieben8" bodies 7 to x (1, 0, 0) y (0, 1, 0) z (0, 0, 1) at (95, -60, 0)
extrude "Extrusion50" cut 1 faces at (94, -116.1667, 27.5) along direction (0, 0, -1) blind 23 on bodies 7 bodies 7
extrude "Extrusion51" add 1 faces at (94, -116.1667, 4.5) along direction (0, 0, 1) blind 2.5 on bodies 7 bodies 7
extrude "Extrusion52" cut 1 faces at (94, -132, 0.3333) along direction (0, 1, 0) blind 12 on bodies 7 bodies 7
copy_body "Körper kopieren/einfügen5" bodies 7 makes body 8
move_body "Verschieben9" bodies 8 to x (1, 0, 0) y (0, 1, 0) z (0, 0, 1) at (29, 0, 0)
copy_body "Körper kopieren/einfügen6" bodies 7 makes body 9
move_body "Verschieben10" bodies 9 to x (1, 0, 0) y (0, 1, 0) z (0, 0, 1) at (57, 0, 0)
extrude "Extrusion53" cut 1 faces at (123, -120, 0.3333) along direction (0, 1, 0) blind 1 on bodies 8 bodies 8
extrude "Extrusion54" cut 1 faces at (151, -120, 0.3333) along direction (0, 1, 0) blind 2 on bodies 9 bodies 9
extrude "Extrusion55" cut 1 faces at (94, -120, 0.3333) along direction (0, 1, 0) blind 2 on bodies 7 bodies 7
extrude "Extrusion56" cut 1 faces at (94, -118, 0.3333) along direction (0, 1, 0) blind 1 on bodies 7 bodies 7
extrude "Extrusion57" add 1 faces at (-2, -72, 7.1667) along direction (0, -1, 0) blind 2.5 on bodies 5 bodies 5
split "Teilen2" by plane through (-2, -51.4, 19.6) normal (0, -1, 0) bodies 5 makes body 10 at (-18.25, -44.8, 14.7) makes body 11 at (-11.005, -52.1994, 2.2667) makes body 12 at (-3, -64.5, -0.3667) makes body 13 at (-11.005, -52.1994, 22.2333)
move_face "Fläche verschieben1" by (0, -2.5, 0) 1 faces at (0, -64.5, -0.3667) on bodies 12
move_body "Verschieben11" bodies 12 to x (1, 0, 0) y (0, 1, 0) z (0, 0, 1) at (0, -2.5, 0)
extrude "Extrusion58" add 3 faces at (-1, -51.4, 2.2667) (-2, -51.4, 9.8) (-2, -51.4, 22.2333) along direction (0, -1, 0) blind 2.5 on bodies 5 bodies 5 12
combine "Kombinieren2" operation add target body 11 tool bodies 5 10 13
extrude "Extrusion59" add 1 faces at (-2, 0, 33.3333) along direction (0, -1, 0) blind 2.5 on bodies 1 bodies 1
split "Teilen3" by plane through (-2, 22.1, 11.6) normal (0, -1, 0) bodies 1 makes body 14 at (-3.6667, 25, 33.3333) makes body 15 at (-11.0199, 19.6017, 7.7333) makes body 16 at (-3, 7.5, 46.1333) makes body 17 at (-11.0199, 19.6017, 42.2667)
move_body "Verschieben12" bodies 16 to x (1, 0, 0) y (0, 1, 0) z (0, 0, 1) at (0, -2.5, 0)
extrude "Extrusion60" add 3 faces at (-2, 22.1, 42.2667) (-2, 22.1, 29.4667) (-2, 22.1, 3.8667) along direction (0, -1, 0) blind 2.5 on bodies 14 bodies 14 16
combine "Kombinieren3" operation add target body 15 tool bodies 1 14 17
copy_body "Körper kopieren/einfügen7" bodies 11 makes body 18
move_body "Verschieben13" bodies 18 to x (1, 0, 0) y (0, 1, 0) z (0, 0, 1) at (0, -50, 0)
extrude "Extrusion61" add 1 faces at (-2, -114.7, 4.9) along direction (0, 0, 1) blind 16 on bodies 18 bodies 18
extrude "Extrusion62" cut 1 faces at (-1, -107.8333, 27.5) along direction (0, 0, -1) blind 5.5 on bodies 18 bodies 18
sketch "Skizze19" plane through (0, 0, 0) normal (1, 0, 0) x (0, 1, 0)
  line L0 (-97, 22) -> (-127, 22)
  line L1 (-127, 22) -> (-127, -3)
  line L2 (-127, -3) -> (-97, -3)
  line L3 (-97, -3) -> (-97, 22)
  line L4 (-127, 22) -> (-97, -3)
  line L5 (-97, 22) -> (-127, -3)
  line L6 (-102, 15.85) -> (-122, 15.85)
  line L7 (-122, 15.85) -> (-122, 3.15)
  line L8 (-122, 3.15) -> (-102, 3.15)
  line L9 (-102, 3.15) -> (-102, 15.85)
  line L10 (-102, 15.85) -> (-122, 3.15) construction
  line L11 (-122, 15.85) -> (-102, 3.15) construction
  point P0 (-112, 9.5)
  dimension "d238" = 20
  dimension "d239" = 12.7
  constraint coincident L0.end L1.start
  constraint coincident L2.end L3.start
  constraint coincident L0.start L3.end
  constraint coincident L1.end L2.start
  constraint horizontal L6
  constraint perpendicular L6 L7
  constraint parallel L6 L8
  constraint parallel L7 L9
  constraint coincident L10 P0
  constraint coincident L11 P0
  constraint midpoint L4 P0
  measures "d238" distance of L7.end L8.end
  measures "d239" distance of L6.end L7.end
extrude "Extrusion63" cut sketch "Skizze19" against normal blind 2.5 contours L4 L5 L6 L8 L9 | L4 L5 L6 | L4 L5 L6 L7 L8 | L4 L5 L8 bodies 18
extrude "Extrusion64" cut 1 faces at (-2.5, -108.6667, 7.3833) along direction (-1, 0, 0) blind 2 on bodies 18 bodies 18
extrude "Extrusion65" add 1 faces at (-18.5, -100.3333, 4.9) along direction (0, 0, 1) blind 15 on bodies 18 bodies 18
extrude "Extrusion66" add 1 faces at (-1, -108.6667, 3.15) along direction (0, 0, 1) blind 15 on bodies 18 bodies 18
extrude "Extrusion67" cut 1 faces at (-1, -53.9, 14.7) along direction (0, 1, 0) blind 0.25 on bodies 11 bodies 11
extrude "Extrusion68" cut 1 faces at (-2, -70.1, 14.7) along direction (0, -1, 0) blind 0.25 on bodies 11 bodies 11
extrude "Extrusion69" add 1 faces at (-22, -48.6667, 16.3333) along direction (-1, 0, 0) blind 8 on bodies 11 bodies 11
extrude "Extrusion70" add 1 faces at (-22, 23.3333, 16.6667) along direction (-1, 0, 0) blind 8 on bodies 15 bodies 15
sketch "Skizze20" plane through (0, 0, 0) normal (0, 0, 1) x (1, 0, 0)
  line L0 (-19, -49.5) -> (-30, -49.5)
  line L1 (-30, -47) -> (-30, -49.5)
  line L2 (-3, -49.5) -> (-3, -77)
  line L3 (-3, -77) -> (0, -77)
  line L4 (-30, -49.5) -> (-3, -77)
  line L5 (-3, -74.1453) -> (-27.1972, -49.5)
  point P0 (-30, -49.5)
  point P1 (-3, -77)
  point P2 (-30, -49.5)
  point P3 (-3, -77)
  dimension "d256" = 2
  constraint coincident P2 P0
  constraint coincident P3 P1
  constraint coincident L2 L5.start
  constraint coincident L0 L5.end
  constraint parallel L4 L5
  measures "d256" distance of L4 L5
extrude "Extrusion71" add sketch "Skizze20" against normal blind 3 bodies 11
extrude "Extrusion72" add 1 faces at (-12, -66.8818, 0) along direction (0, 0, 1) blind 4.9 on bodies 11 bodies 11
extrude "Extrusion73" add 1 faces at (-12, -66.8818, 4.9) along direction (0, 0, 1) blind 7.9 from surface at 14.7 on bodies 11 bodies 11
sketch "Skizze21" plane through (0, 0, 0) normal (0, 0, 1) x (1, 0, 0)
  line L0 (-19, 22.5) -> (-30, 22.5)
  line L1 (-30, 25) -> (-30, 22.5)
  line L2 (-3, 22.5) -> (-3, -5)
  line L3 (-3, -5) -> (0, -5)
  line L4 (-3, -5) -> (-30, 22.5)
  line L5 (-27.1972, 22.5) -> (-3, -2.1453)
  point P0 (-30, 22.5)
  point P1 (-30, 22.5)
  point P2 (-3, -5)
  point P3 (-3, -5)
  dimension "d264" = 2
  constraint coincident P3 P2
  constraint coincident P1 P0
  constraint coincident L0 L5.start
  constraint coincident L2 L5.end
  constraint parallel L4 L5
  measures "d264" distance of L4 L5
extrude "Extrusion74" add sketch "Skizze21" along normal blind 11.6 bodies 15
extrude "Extrusion75" add 1 faces at (-12, 5.1182, 11.6) along direction (0, 0, 1) blind 11.6 from surface at 26.8 on bodies 15 bodies 15
split "Teilen4" by plane through (-19, 27.3, 0) normal (0, -1, 0) bodies 15 makes body 19 at (-19.75, 28.05, 16.6667) makes body 20 at (0, 6.8, 46.1333)
delete_body "Körper entfernen1" bodies 2
delete_body "Körper entfernen2" bodies 6
combine "Kombinieren4" operation add target body 15 tool bodies 20 19
extrude "Extrusion76" cut sketch "Skizze19" against normal blind 10 contours L4 L5 L6 L8 L9 | L4 L5 L6 | L4 L5 L6 L7 L8 | L4 L5 L8 bodies 18
extrude "Extrusion9" [rolled back] along distance -50 taper angle 0
extrude "Extrusion10" [suppressed]
extrude "Extrusion11" [rolled back] along distance -8 taper angle 0
equation "d7 = ( 13.4 / 2 ) * 1 mm"
equation "d8 = ( 13.4 / 2 ) * 1 mm"
equation "d181 = 19.6 mm - 4.9 mm"
equation "d236 = -30.5 mm + 25 mm"
